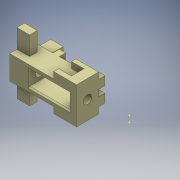
# Autodesk Inventor part: negyszogletes_teszt_v2_1064um
Saved by Autodesk Inventor 2016 (Build 200138000, 138)
## iProperties
Created: 2015-10-07
Part Number: negyszogletes_teszt_v2_1064um
Material: Polypropylene
Document SubType Name: Modeling
Designer: Tony
Density: 0.899 g/cm^3
Appearance: Smooth - Ash
Mass: 0.172809 g
Surface Area: 5.52049 cm^2
Volume: 0.192224 cm^3
Author: Tony
Autodesk Inventor part; units mm, degrees
ref_plane "YZ Plane" through (0, 0, 0) normal (1, 0, 0) x (0, 1, 0)
ref_plane "XZ Plane" through (0, 0, 0) normal (0, 1, 0) x (-1, 0, 0)
ref_plane "XY Plane" through (0, 0, 0) normal (0, 0, 1) x (1, 0, 0)
sketch "Sketch1" plane through (0, 0, 0) normal (0, 1, 0) x (-1, 0, 0)
  line L0 (9, -13.6) -> (17, -13.6)
  line L1 (17, -13.6) -> (17, -17.4)
  line L2 (17, -17.4) -> (9, -17.4)
  line L3 (9, -17.4) -> (9, -13.6)
  line L4 (16, -14.3) -> (10, -14.3)
  line L5 (10, -14.3) -> (10, -16.7)
  line L6 (10, -16.7) -> (16, -16.7)
  line L7 (16, -16.7) -> (16, -14.3)
  dimension "d12" = 6
  dimension "d13" = 8
  dimension "d14" = 1
  dimension "d15" = 2.4
  dimension "d16" = 0.7
  dimension "d17" = 0.7
  constraints: 16 end point, 4 parallel, 2 horizontal, 2 perpendicular
  measures "d12" distance of L4.start L4.end
  measures "d13" distance between parallel lines of L3 L1
  measures "d14" distance between parallel lines of L3 L5
  measures "d15" distance of L6.end L4.start
  measures "d16" distance between parallel lines of L4 L0
  measures "d17" distance between parallel lines of L2 L6
extrude "Extrusion1" add sketch "Sketch1" along normal blind 3.5 contours L0 L1 L2 L3 | L7 L6 L5 L4
extrude "Extrusion2" cut sketch "Sketch1" along normal blind 2.8 contours L7 L6 L5 L4
hole "Hole3" at (-17, 1.75, -15.5) direction (1, 0, 0) diameter 1.35 end through all
sketch "Sketch5" plane through (-17, 0, -17.4) normal (-1, 0, 0) x (0, 0, 1)
  line L0 (3.8, 3.5) -> (0, 3.5)
  line L1 (0, 3.5) -> (0, 0)
  line L2 (0, 0) -> (3.8, 0)
  line L3 (3.8, 0) -> (3.8, 3.5)
  line L4 (3.8, 0) -> (0, 0) projected
  line L5 (0, 0) -> (-0.8, 0)
  line L6 (0, 1.2) -> (0, 0)
  line L7 (0, 0) -> (0, 3.5) projected
  line L8 (0, 1.15) -> (-3, 1.15)
  line L9 (-3, 1.15) -> (-3, 2.35)
  line L10 (-3, 2.35) -> (0, 2.35)
  line L11 (0, 2.35) -> (0, 1.15)
  line L12 (3.8, 0) -> (3.8, 3.5) projected
  line L13 (3.8, 1.2) -> (3.8, 0)
  line L14 (3.8, 1.15) -> (6.8, 1.15)
  line L15 (6.8, 1.15) -> (6.8, 2.35)
  line L16 (6.8, 2.35) -> (3.8, 2.35)
  line L17 (3.8, 2.35) -> (3.8, 1.15)
  line L18 (0, 3.5) -> (3.8, 3.5) projected
  line L19 (2.5, 3.5) -> (1.3, 3.5)
  line L20 (1.3, 3.5) -> (1.3, 6.5)
  line L21 (1.3, 6.5) -> (2.5, 6.5)
  line L22 (2.5, 6.5) -> (2.5, 3.5)
  line L23 (0.2329, 3.5) -> (1.4329, 3.5)
  point P0 (17.4, 0)
  dimension "d109" = 1.2
  dimension "d111" = 1.2
  dimension "d112" = 3
  dimension "d131" = 3
  dimension "d132" = 3
  dimension "d133" = 1.15
  dimension "d134" = 1.3
  constraints: 40 end point, 8 parallel, 6 horizontal, 6 point on line, 4 perpendicular, 1 collinear
  measures "d109" distance of L8.end L9.end
  measures "d111" distance of L20.end L21.end
  measures "d112" distance of L19.end L20.end
  measures "d131" distance of L8.start L8.end
  measures "d132" distance of L15.end L16.end
  measures "d133" distance from line of L23.start L10
  measures "d134" distance between parallel lines of L12 L22
extrude "Extrusion4" add sketch "Sketch5" along normal blind 2
hole "Hole8" at (-17, 1.75, -15.5) direction (-1, 0, 0) diameter 2.5 end through all
sketch "Sketch7" plane through (-9, 0, -17.4) normal (0, 0, -1) x (-1, 0, 0)
  line L0 (0, 0) -> (0, 3.5) projected
  line L1 (0, 3.5) -> (10, 3.5) projected
  line L2 (0, 0) -> (3, 0)
  line L3 (3, 0) -> (3, 3.5)
  line L4 (3, 3.5) -> (0, 3.5)
  line L5 (0, 3.5) -> (0, 0)
  line L6 (3, 0.8155) -> (1, 0.8155)
  line L7 (1, 0.8155) -> (1, 2.8155)
  line L8 (1, 2.8155) -> (3, 2.8155)
  line L9 (3, 2.8155) -> (3, 0.8155)
  point P0 (-9, 0)
  dimension "d135" = 3
  dimension "d136" = 2
  dimension "d137" = 2
  constraints: 16 end point, 4 parallel, 2 horizontal, 2 perpendicular, 1 point on line
  measures "d135" distance of L4.end L3.end
  measures "d136" distance of L7.end L8.end
  measures "d137" distance of L6.end L7.end
extrude "Extrusion6" add sketch "Sketch7" along normal blind 1 contours L0 L1 L3 L8 L7 L6 L2
sketch "Sketch8" plane through (0, 3.5, 0) normal (0, 1, 0) x (1, 0, 0)
  line L0 (-12, 17.4) -> (-10, 17.4) projected
  line L1 (-9, 13.6) -> (-19, 13.6) projected
  line L2 (-12, 17.4) -> (-9, 17.4)
  line L3 (-9, 17.4) -> (-9, 13.6)
  line L4 (-9, 13.6) -> (-12, 13.6)
  line L5 (-12, 13.6) -> (-12, 17.4)
  line L6 (-12, 16.5) -> (-10, 16.5)
  line L7 (-10, 16.5) -> (-10, 14.5)
  line L8 (-10, 14.5) -> (-12, 14.5)
  line L9 (-12, 14.5) -> (-12, 16.5)
  line L10 (-10, 14.3) -> (-10, 16.7) projected
  line L11 (-10, 16) -> (-9, 16)
  line L12 (-9, 16) -> (-9, 15)
  line L13 (-9, 15) -> (-10, 15)
  line L14 (-10, 15) -> (-10, 16)
  point P0 (0, 0)
  point P1 (-2, 17.4)
  dimension "d140" = 2
  dimension "d141" = 2
  dimension "d142" = 0.9
  dimension "d143" = 1
  dimension "d144" = 0.5
  constraints: 24 end point, 6 parallel, 3 horizontal, 3 perpendicular, 2 point on line
  measures "d140" distance of L7.end L8.end
  measures "d141" distance of L6.end L7.end
  measures "d142" distance between parallel lines of L1 L8
  measures "d143" distance between parallel lines of L11 L13
  measures "d144" distance between parallel lines of L8 L13
extrude "Extrusion7" add sketch "Sketch8" along normal blind 1 contours L0 L2 L3 L11 L7 L6 L5 | L8 L7 L13 L3 L1 L5
sketch "Sketch9" plane through (0, 3.5, 0) normal (0, 1, 0) x (1, 0, 0)
  line L0 (-19, 17.4) -> (-12, 17.4) projected
  line L1 (-12, 13.6) -> (-19, 13.6) projected
  line L2 (-14.6468, 17.4) -> (-15.6468, 17.4)
  line L3 (-15.6468, 17.4) -> (-15.6468, 13.6)
  line L4 (-15.6468, 13.6) -> (-14.6468, 13.6)
  line L5 (-14.6468, 13.6) -> (-14.6468, 17.4)
  line L6 (-14.6468, 16) -> (-15.6468, 16)
  line L7 (-15.6468, 16) -> (-15.6468, 15)
  line L8 (-15.6468, 15) -> (-14.6468, 15)
  line L9 (-14.6468, 15) -> (-14.6468, 16)
  point P0 (0, 0)
  dimension "d147" = 1
  dimension "d148" = 1
  dimension "d149" = 1.4
  constraints: 16 end point, 4 parallel, 2 horizontal, 2 perpendicular, 2 point on line
  measures "d147" distance of L4.end L3.end
  measures "d148" distance between parallel lines of L8 L6
  measures "d149" distance between parallel lines of L1 L8
extrude "Extrusion8" add sketch "Sketch9" along normal blind 1 contours L0 L5 L6 L3 | L8 L5 L1 L3
sketch "Sketch10" plane through (-19, 0, -13.6) normal (0, 0, 1) x (1, 0, 0)
  line L0 (7, 3.5) -> (7, 4.5) projected
  line L1 (7, 3.5) -> (10, 3.5)
  line L2 (10, 3.5) -> (10, 0)
  line L3 (10, 0) -> (7, 0)
  line L4 (7, 0) -> (7, 3.5)
  line L5 (7, 2.8) -> (9, 2.8)
  line L6 (9, 2.8) -> (9, 0.8)
  line L7 (9, 0.8) -> (7, 0.8)
  line L8 (7, 0.8) -> (7, 2.8)
  point P0 (19, 0)
  dimension "d152" = 2
  dimension "d153" = 2
  dimension "d154" = 0.8
  constraints: 16 end point, 4 parallel, 2 horizontal, 2 perpendicular, 1 point on line
  measures "d152" distance of L6.end L7.end
  measures "d153" distance of L5.end L6.end
  measures "d154" distance between parallel lines of L3 L7
extrude "Extrusion9" add sketch "Sketch10" along normal blind 1 contours L1 L2 L3 L4 L7 L6 L5
chamfer "Chamfer4" distance 0.2 angle 45 2 edges at (-13, 0, -14.3) (-13, 0, -16.7)
thicken "Thicken4" operation add thickness 0.6 both sides no extend neighbours yes toward (1, 0, 0) faces at (-9, 1.75, -13.3417)
thicken "Thicken5" operation add thickness 0.6 both sides no extend neighbours yes toward (1, 0, 0) faces at (-10, 0.4933, -15.4729)
sketch "Sketch11" plane through (-19, 0, -12.6) normal (0, 0, 1) x (1, 0, 0)
  point P0 (19, 0)
sketch "Sketch12" plane through (-19, 0, -12.6) normal (0, 0, 1) x (1, 0, 0)
  point P0 (19, 0)
sketch "Sketch13" plane through (-19, 2.35, -13.6) normal (0, 0, 1) x (1, 0, 0)
  point P0 (19, -2.35)
body "Solid1"
